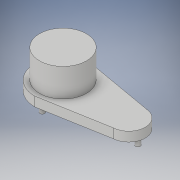
# Autodesk Inventor part: LIDAR-Sensor
Saved by Autodesk Inventor 2019.5 (Build 235369000, 369)
## iProperties
Created: 2021-10-01
Part Number: LIDAR-Sensor
Material: Generisch
Document SubType Name: Modeling
Designer: mritt
Density: 1 g/cm^3
Appearance: Vorgabe
Author: mritt
Autodesk Inventor part; units mm, degrees
ref_plane "YZ Plane" through (0, 0, 0) normal (1, 0, 0) x (0, 1, 0)
ref_plane "XZ Plane" through (0, 0, 0) normal (0, 1, 0) x (-1, 0, 0)
ref_plane "XY Plane" through (0, 0, 0) normal (0, 0, 1) x (1, 0, 0)
sketch "Skizze1" plane through (0, 0, 0) normal (0, 1, 0) x (-1, 0, 0)
  circle A0 centre (9.2308, -70.3479) radius 17.5
  arc A1 (79.2308, -100.3479) -> (79.2308, -40.3479) centre (79.2308, -70.3479) ccw
  line L0 (79.2308, -40.3479) -> (8.002, -52.8911)
  line L1 (79.2308, -100.3479) -> (7.9966, -87.8043)
  circle A2 centre (79.2308, -70.3479) radius 20
  point P0 (0, 0)
  dimension "d1" = 35
  dimension "d20" = 30
  dimension "d21" = 70
  dimension "d22" = 0
  dimension "d24" = 40
  constraints: 4 end point, 4 point on circle, 3 centre point, 1 coincident
  measures "d1" diameter of A0
  measures "d20" radius of A1
  measures "d21" distance of A1.centre A0.centre
  measures "d22" vertical distance of A1.centre A0.centre
  measures "d24" diameter of A2
extrude "Extrusion1" add sketch "Skizze1" along normal blind 10 contours A0 | A0 L0 A1 L1 | A2
sketch "Skizze2" plane through (0, 10, 0) normal (0, 1, 0) x (1, 0, 0)
  arc A0 (-79.2308, 100.3479) -> (-79.2308, 40.3479) centre (-79.2308, 70.3479) ccw projected
  circle A1 centre (-79.2308, 70.3479) radius 25
  point P0 (0, 0)
  dimension "d23" = 50
  constraints: 1 centre point, 1 coincident
  measures "d23" diameter of A1
extrude "Extrusion2" add sketch "Skizze2" along normal blind 30
sketch "Skizze3" plane through (0, 0, 0) normal (0, -1, 0) x (1, 0, 0)
  circle A0 centre (-79.56, -89.4817) radius 2.5
  circle A1 centre (-80.4525, -49.4817) radius 2.5
  circle A2 centre (0.7692, -70.1017) radius 2.5
  arc A3 (-8.002, -52.8911) -> (-8.002, -52.8911) centre (-9.2308, -70.3479) ccw projected
  point P0 (0, 0)
  point P1 (-8.4112, -91.1215)
  point P2 (-79.56, -69.4817)
  dimension "d7" = 5
  dimension "d8" = 5
  dimension "d9" = 5
  dimension "d10" = 10
  dimension "d11" = 20
  dimension "d12" = 0
  dimension "d13" = 20
  constraints: 3 centre point, 1 other
  measures "d7" diameter of A0
  measures "d8" diameter of A1
  measures "d9" diameter of A2
  measures "d10" horizontal distance of point (-9.231, -70.348) A2.centre
  measures "d11" distance of point (-79.56, -69.482) A0.centre
  measures "d12" horizontal distance of point (-79.56, -69.482) A0.centre
  measures "d13" vertical distance of point (-79.56, -69.482) A1.centre
extrude "Extrusion3" add sketch "Skizze3" along normal blind 10 contours A0 | A1 | A2
